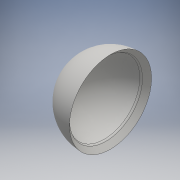
# Autodesk Inventor part: tomato2016
Saved by Autodesk Inventor 2016 (Build 200138000, 138)
## iProperties
Created: 2016-05-04
Part Number: tomato2016
Material: 一般
Document SubType Name: Modeling
Designer: 宏太
Density: 1 g/cm^3
Appearance: 既定
Author: 宏太
Autodesk Inventor part; units mm, degrees
ref_plane "YZ Plane" through (0, 0, 0) normal (1, 0, 0) x (0, 1, 0)
ref_plane "XZ Plane" through (0, 0, 0) normal (0, 1, 0) x (-1, 0, 0)
ref_plane "XY Plane" through (0, 0, 0) normal (0, 0, 1) x (1, 0, 0)
sketch "スケッチ1" plane through (0, 0, 0) normal (0, 1, 0) x (-1, 0, 0)
  arc A0 (25, 0) -> (0, 25) centre (0, 0) ccw
  line L0 (0, 25) -> (3.213, 21.7641)
  arc A1 (22, 0) -> (3.213, 21.7641) centre (0, 0) ccw
  line L1 (25, 0) -> (22, 0)
  point P0 (0, 0)
  dimension "d0" = 25
  dimension "d1" = 25
  dimension "d2" = 25
  dimension "d4" = 22
  constraints: 4 end point, 4 point on circle, 2 centre point, 1 horizontal
  measures "d0" distance of point (0, 0) L1.start
  measures "d1" distance of point (0, 0) L0.start
  measures "d2" radius of A0
  measures "d4" distance of A0.centre L1.end
revolve "回転1" add sketch "スケッチ1" angle 360 about axis through (-25, 0, 0) along (1, 0, 0)
fillet "フィレット1" radius 2 1 edges at (-3.213, 0, -21.7641)
